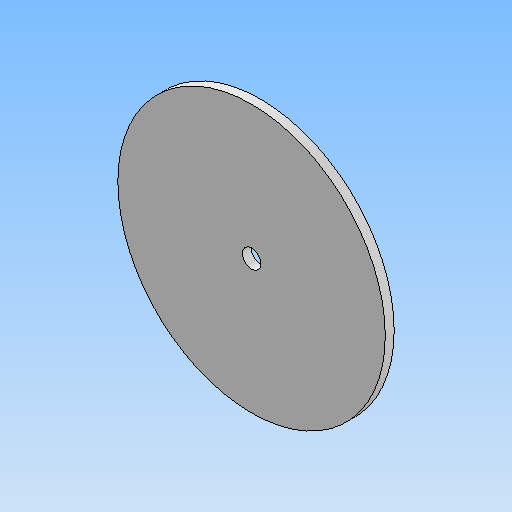
# Autodesk Inventor part: CRA-1027
Saved by Autodesk Inventor 2025.4 (Build 294407000, 407)
## iProperties
RuleStatus: InUse
Created: 2025-12-20
Part Number: CRA-1027
Material: Steel, Mild
Document SubType Name: Sheet Metal
Designer: josh
Mass: 11360 g
Surface Area: 2441.73 cm^2
Volume: 1447.14 cm^3
Density: 7.85 g/cm^3
Flat Pattern Width: 38.1795 cm
Flat Pattern Length: 38.1795 cm
Flat Pattern Area: 1457.67 cm^2
Sheet Metal Rule: Mild Steel .5
Sheet Metal Width: 15.031 in
Sheet Metal Length: 15.031 in
Sheet Metal Area: 225.940 in^2
Appearance: Default
Description: 25Lb Counter Weight Plate
AfterDocOpen0: PartNumber
Flat pattern length: =<Sheet Metal Length>
Flat pattern width: =<Sheet Metal Width>
Thickness: 0.500 in
Qty: 1
Flat Length: 15.0313
Flat Width: 15.0313
Part Area: 225.93997969
Author: josh
Autodesk Inventor part; units mm, degrees
ref_plane "YZ Plane" through (0, 0, 0) normal (1, 0, 0) x (0, 1, 0)
ref_plane "XZ Plane" through (0, 0, 0) normal (0, 1, 0) x (-1, 0, 0)
ref_plane "XY Plane" through (0, 0, 0) normal (0, 0, 1) x (1, 0, 0)
sketch "Sketch12" plane through (0, 0, 0) normal (0, 0, 1) x (1, 0, 0)
  circle A0 centre (0, 0) radius 190.8975
  circle A1 centre (0, 0) radius 13.081
  dimension "d107" = 381.795
  dimension "d108" = 26.162
  measures "d107" diameter of A0
  measures "d108" diameter of A1
extrude "Plate4" add sketch "Sketch12" along normal blind 12.7
equation "\"d109\" = Thickness"
equation "\"BendRadius\" = Thickness"
equation "\"BendReliefWidth\" = Thickness"
equation "\"BendReliefDepth\" = 0.5 * Thickness"
equation "\"CornerReliefSize\" = 4 * Thickness"
equation "\"MinimumRemnant\" = 2 * Thickness"
equation "\"TransitionRadius\" = BendRadius"
equation "\"JacobiRadiusSize\" = BendRadius"
equation "\"GapSize\" = Thickness"
equation "\"Thickness\" = 12.7"
body "Solid3"
